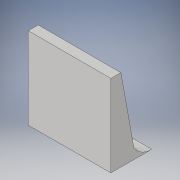
# Autodesk Inventor part: palm_side_plate
Saved by Autodesk Inventor 2019 (Build 230136000, 136)
## iProperties
Created: 2024-08-27
Part Number: palm_side_plate
Material: Generisch
Document SubType Name: Modeling
Designer: nic
Density: 1 g/cm^3
Appearance: Vorgabe
Author: nic
Autodesk Inventor part; units mm, degrees
ref_plane "YZ Plane" through (0, 0, 0) normal (1, 0, 0) x (0, 1, 0)
ref_plane "XZ Plane" through (0, 0, 0) normal (0, 1, 0) x (-1, 0, 0)
ref_plane "XY Plane" through (0, 0, 0) normal (0, 0, 1) x (1, 0, 0)
ref_plane "Arbeitsebene1" through (0, 0, 32) normal (0, 0, 1) x (1, 0, 0)
sketch "Skizze1" plane through (0, 0, 32) normal (0, 0, 1) x (1, 0, 0)
  line L0 (0, -2) -> (-10.2, -2) construction
  line L1 (0, 0) -> (-10.2, 0) construction
  line L2 (0, 0) -> (0, -2) construction
  line L3 (-10.2, 0) -> (-10.2, -2) construction
  line L4 (-10.2, -2) -> (-0.1, -2)
  line L5 (-0.1, -2) -> (-0.1, 8)
  line L6 (-0.1, 8) -> (-10.2, 8)
  line L7 (-10.2, 8) -> (-10.2, -2)
  dimension "d0" = 10.1
  dimension "d1" = 10
  constraints: 8 end point, 2 parallel, 1 horizontal, 1 perpendicular
  measures "d0" distance of L6.end L5.end
  measures "d1" distance of L5.end L4.end
extrude "Extrusion1" add sketch "Skizze1" along normal blind 5
sketch "Skizze2" plane through (-0.1, -2, 32) normal (1, 0, 0) x (0, 0, -1)
  line L0 (-3.3973, 7.8087) -> (-3.7161, 9.6721) projected
  line L1 (-3.0763, 5.9578) -> (-2.8181, 4.4664) projected
  line L2 (-2.7379, 2.2485) -> (-2.2681, 1.397) construction
  line L3 (-1.7937, 0.8596) -> (-2.122, 0.4) construction
  line L4 (-2.7257, 0.0358) -> (-1.7762, -0.6392) construction
  line L5 (0, 0) -> (0, 10) construction
  line L6 (0, 10) -> (-5, 10) construction
  line L7 (-5, 0) -> (-5, 10) construction
  line L8 (0, 0) -> (-5, 0) construction
  line L9 (0, 10) -> (-5, 10) construction
  line L10 (-3.7764, 10) -> (-2.1928, 1.2606)
  line L11 (-1.7937, 0.8596) -> (-2.122, 0.4) projected
  line L12 (-2.6421, 0.9776) -> (-2.2681, 1.397) construction
  line L13 (-2.122, 0.4) -> (-2.1571, -0.2183) construction
  line L14 (-1.7937, 0.8596) -> (-2.122, 0.4) projected
  line L15 (-1.7937, 0.8596) -> (-2.122, 0.4) projected
  arc A0 (-2.1928, 1.2606) -> (0, 0) centre (0, 2.5375) ccw
  line L16 (-3.7764, 10) -> (0, 10)
  line L17 (0, 10) -> (0, 0)
  point P0 (32, 2)
  point P1 (0.0012, 1.774)
  constraints: 6 end point, 2 point on circle, 2 point on line, 1 centre point, 1 horizontal, 1 perpendicular, 1 tangent, 1 other
extrude "Extrusion2" cut sketch "Skizze2" against normal through all
